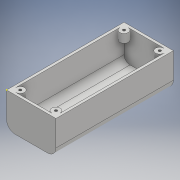
# Autodesk Inventor part: ICE CREAM
Saved by Autodesk Inventor 2017 (Build 210142000, 142)
## iProperties
Created: 2019-09-14
Part Number: ICE CREAM
Material: Generic
Document SubType Name: Modeling
Designer: Admin
Density: 1 g/cm^3
Appearance: Default
Mass: 66.2599 g
Surface Area: 446.005 cm^2
Volume: 66.2599 cm^3
Author: Admin
Autodesk Inventor part; units mm, degrees
ref_plane "YZ Plane" through (0, 0, 0) normal (1, 0, 0) x (0, 1, 0)
ref_plane "XZ Plane" through (0, 0, 0) normal (0, 1, 0) x (-1, 0, 0)
ref_plane "XY Plane" through (0, 0, 0) normal (0, 0, 1) x (1, 0, 0)
sketch "Sketch1" plane through (0, 0, 0) normal (0, 0, 1) x (1, 0, 0)
  line L0 (0, 0) -> (58, 0)
  line L1 (58, 0) -> (58, 138)
  line L2 (58, 138) -> (0, 138)
  line L3 (0, 138) -> (0, 0)
  dimension "d0" = 58
  dimension "d1" = 138
  constraints: 8 end point, 3 perpendicular, 1 horizontal
  measures "d0" distance of L0.start L0.end
  measures "d1" distance of L0.end L1.end
extrude "Extrusion1" add sketch "Sketch1" along normal blind 40
fillet "Fillet1" radius 10 2 edges at (0, 69, 0) (58, 69, 0)
shell "Shell1" thickness 3 removed faces 1 at (19.3333, 92, 40)
sketch "Sketch2" plane through (0, 0, 40) normal (0, 0, 1) x (1, 0, 0)
  line L0 (55, 135) -> (55, 3) projected
  line L1 (55, 135) -> (55, 130)
  line L2 (55, 130) -> (50, 130)
  circle A0 centre (50, 130) radius 5
  point P0 (0, 0)
  dimension "d6" = 5
  dimension "d7" = 5
  constraints: 4 end point, 1 coincident, 1 horizontal, 1 horizontal alignment, 1 point on line, 2 other
  measures "d6" distance of L0.start L1.end
  measures "d7" distance of L1.end L2.end
extrude "Extrusion3" add sketch "Sketch2" against normal blind 10
sketch "Sketch10" plane through (0, 0, 40) normal (0, 0, 1) x (1, 0, 0)
  line L0 (3, 135) -> (50, 135) projected
  line L1 (48, 135) -> (55, 135) projected
  line L2 (50, 135) -> (55, 135)
  arc A0 (55, 130) -> (50, 135) centre (50, 130) ccw projected
  line L3 (55, 135) -> (50, 135)
  line L4 (55, 135) -> (55, 3) projected
  line L5 (55, 135) -> (55, 130)
  point P0 (0, 0)
  constraints: 6 end point, 2 collinear, 2 tangent
extrude "Extrusion4" add sketch "Sketch10" against normal blind 10
sketch "Sketch11" plane through (0, 0, 40) normal (0, 0, 1) x (1, 0, 0)
  arc A0 (55, 130) -> (50, 135) centre (50, 130) ccw projected
  circle A1 centre (50, 130) radius 1.5
  point P0 (0, 0)
  dimension "d14" = 3
  constraints: 1 centre point, 1 coincident
  measures "d14" diameter of A1
extrude "Extrusion5" cut sketch "Sketch11" against normal blind 5
thread "Thread1" size "M3x0.5" class "6H" standard "ANSI Metric M Profile" full length
sketch "Sketch12" plane through (0, 0, 40) normal (0, 0, 1) x (1, 0, 0)
  line L0 (3, 3) -> (3, 135) projected
  line L1 (55, 3) -> (3, 3) projected
  line L2 (3, 3) -> (3, 8)
  line L3 (3, 8) -> (8, 8)
  line L4 (10, 138) -> (10, 0) projected
  circle A0 centre (8, 8) radius 5
  point P0 (0, 0)
  dimension "d20" = 5
  dimension "d21" = 5
  constraints: 4 end point, 1 coincident, 1 horizontal alignment, 1 perpendicular, 1 point on line, 2 other
  measures "d20" distance of L0.start L2.end
  measures "d21" distance of L2.end L3.end
extrude "Extrusion6" add sketch "Sketch12" against normal blind 10 contours A0 L4 | A0 L4
sketch "Sketch15" plane through (0, 0, 40) normal (0, 0, 1) x (1, 0, 0)
  line L0 (8, 3) -> (3, 3) projected
  line L1 (3, 3) -> (3, 135) projected
  line L2 (8, 3) -> (3, 3)
  arc A0 (3, 8) -> (8, 3) centre (8, 8) ccw projected
  line L3 (3, 3) -> (8, 3)
  point P0 (0, 0)
  constraints: 4 end point, 1 perpendicular, 1 tangent
extrude "Extrusion7" add sketch "Sketch15" against normal blind 10
sketch "Sketch16" plane through (0, 0, 40) normal (0, 0, 1) x (1, 0, 0)
  arc A0 (8, 3) -> (3, 8) centre (8, 8) ccw projected
  circle A1 centre (8, 8) radius 1.5
  point P0 (0, 0)
  dimension "d26" = 3
  constraints: 1 centre point, 1 coincident
  measures "d26" diameter of A1
extrude "Extrusion8" cut sketch "Sketch16" against normal blind 5
thread "Thread2" size "M3x0.5" class "6H" standard "ANSI Metric M Profile" full length
sketch "Sketch17" plane through (0, 0, 40) normal (0, 0, 1) x (1, 0, 0)
  line L0 (10, 138) -> (10, 0) projected
  line L1 (8, 135) -> (8, 130)
  circle A0 centre (8, 130) radius 5
  point P0 (0, 0)
  point P1 (3, 135)
  dimension "d31" = 5
  dimension "d32" = 5
  constraints: 2 end point, 1 coincident, 1 parallel, 1 vertical alignment, 2 other
  measures "d31" distance of point (3, 135) L1.start
  measures "d32" distance of L1.start L1.end
extrude "Extrusion9" add sketch "Sketch17" against normal blind 10
sketch "Sketch18" plane through (0, 0, 40) normal (0, 0, 1) x (1, 0, 0)
  arc A0 (8, 135) -> (3, 130) centre (8, 130) ccw projected
  line L0 (3, 3) -> (3, 135) projected
  line L1 (8, 135) -> (3, 135)
  line L2 (3, 135) -> (8, 135)
  line L3 (3, 135) -> (10, 135) projected
  point P0 (0, 0)
  constraints: 4 end point, 1 collinear
extrude "Extrusion10" add sketch "Sketch18" against normal blind 10
sketch "Sketch19" plane through (0, 0, 40) normal (0, 0, 1) x (1, 0, 0)
  arc A0 (3, 130) -> (8, 135) centre (8, 130) ccw projected
  circle A1 centre (8, 130) radius 1.5
  point P0 (0, 0)
  dimension "d37" = 3
  constraints: 1 centre point, 1 coincident
  measures "d37" diameter of A1
extrude "Extrusion11" cut sketch "Sketch19" against normal blind 5
thread "Thread3" size "M3x0.5" class "6H" standard "ANSI Metric M Profile" full length
sketch "Sketch21" plane through (0, 0, 40) normal (0, 0, 1) x (1, 0, 0)
  circle A0 centre (50, 8) radius 5
  point P0 (0, 0)
  point P1 (55, 3)
  constraints: 1 centre point
extrude "Extrusion12" add sketch "Sketch21" against normal blind 10
sketch "Sketch23" plane through (0, 0, 40) normal (0, 0, 1) x (1, 0, 0)
  arc A0 (50, 3) -> (55, 8) centre (50, 8) ccw projected
  line L0 (55, 135) -> (55, 3) projected
  line L1 (50, 3) -> (55, 3)
  line L2 (55, 3) -> (50, 3) projected
  line L3 (55, 3) -> (50, 3)
  point P0 (0, 0)
  constraints: 4 end point, 1 collinear
extrude "Extrusion13" add sketch "Sketch23" against normal blind 10
sketch "Sketch24" plane through (0, 0, 40) normal (0, 0, 1) x (1, 0, 0)
  arc A0 (55, 8) -> (50, 3) centre (50, 8) ccw projected
  circle A1 centre (50, 8) radius 1.5
  point P0 (0, 0)
  dimension "d48" = 3
  constraints: 1 centre point, 1 coincident
  measures "d48" diameter of A1
extrude "Extrusion14" cut sketch "Sketch24" against normal blind 5
thread "Thread4" size "M3x0.5" class "6H" standard "ANSI Metric M Profile" full length
sketch "Sketch25" plane through (0, 0, 40) normal (0, 0, 1) x (1, 0, 0)
  point P0 (0, 0)
body "Solid1"
